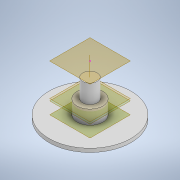
# Autodesk Inventor part: mold
Saved by Autodesk Inventor 2021 (Build 250183000, 183)
## iProperties
Created: 2020-07-07
Part Number: mold
Material: Generic
Document SubType Name: Modeling
Designer: adaml
Density: 1 g/cm^3
Appearance: Default
Author: adaml
Autodesk Inventor part; units mm, degrees
ref_plane "YZ Plane" through (0, 0, 0) normal (1, 0, 0) x (0, 1, 0)
ref_plane "XZ Plane" through (0, 0, 0) normal (0, 1, 0) x (-1, 0, 0)
ref_plane "XY Plane" through (0, 0, 0) normal (0, 0, 1) x (1, 0, 0)
ref_plane "Work Plane3" through (0, 0, 0) normal (0, -1, 0) x (1, 0, 0)
sketch "Sketch2" plane through (0, 0, 0) normal (0, -1, 0) x (1, 0, 0)
  circle A0 centre (0, 0) radius 22.352
  arc A1 (22.352, 0) -> (-22.352, 0) centre (0, 0) ccw projected
  line L0 (22.352, 0) -> (-22.352, 0)
  constraints: 2 end point, 1 centre point, 1 coincident, 1 horizontal
extrude "Extrusion2" add sketch "Sketch2" along normal blind 2
ref_plane "Work Plane5" through (0, 0, 0) normal (0, 1, 0) x (1, 0, 0)
sketch "Sketch3" plane through (0, 0, 0) normal (0, 1, 0) x (1, 0, 0)
  circle A0 centre (0, 0) radius 7
  line L0 (-20.955, 0) -> (20.955, 0) projected
  line L1 (-7, 0) -> (7, 0)
  dimension "d6" = 14
  constraints: 2 end point, 2 point on circle, 2 point on line, 1 centre point, 1 coincident
  measures "d6" diameter of A0
extrude "Extrusion3" add sketch "Sketch3" along normal blind 7.62
ref_plane "Work Plane4" through (0, -2, 0) normal (0, -1, 0) x (1, 0, 0)
sketch "Sketch4" plane through (0, -2, 0) normal (0, -1, 0) x (1, 0, 0)
  circle A0 centre (0, 0) radius 6
  dimension "d9" = 12
  constraints: 1 centre point, 1 coincident
  measures "d9" diameter of A0
extrude "Extrusion4" cut sketch "Sketch4" against normal blind 8.5725
ref_plane "Work Plane6" through (0, 7.62, 0) normal (0, 1, 0) x (1, 0, 0)
sketch "Sketch5" plane through (0, 7.62, 0) normal (0, 1, 0) x (1, 0, 0)
  circle A0 centre (0, 0) radius 4
  line L0 (7, 0) -> (-7, 0) projected
  line L1 (4, 0) -> (-4, 0)
  dimension "d12" = 8
  constraints: 2 end point, 2 point on circle, 2 point on line, 1 centre point, 1 coincident
  measures "d12" diameter of A0
extrude "Extrusion5" add sketch "Sketch5" along normal blind 10.16
ref_plane "Work Plane7" through (0, 6.5725, 0) normal (0, -1, 0) x (1, 0, 0)
sketch "Sketch6" plane through (0, 6.5725, 0) normal (0, -1, 0) x (1, 0, 0)
  circle A0 centre (0, 0) radius 3
  dimension "d15" = 6
  constraints: 1 centre point, 1 coincident
  measures "d15" diameter of A0
extrude "Extrusion6" cut sketch "Sketch6" against normal blind 10.16
ref_plane "Work Plane1" through (0, 25.4, 0) normal (0, 1, 0) x (1, 0, 0)
sketch "Sketch7" plane through (0, 25.4, 0) normal (0, 1, 0) x (1, 0, 0)
  point P0 (0, 0)
ref_plane "Work Plane2" through (0, 25.4, 0) normal (0, 1, 0) x (1, 0, 0)
sketch "Sketch12" plane through (0, 25.4, 0) normal (0, 1, 0) x (1, 0, 0)
  circle A0 centre (0, 0) radius 16.1182
  circle A1 centre (0, 0) radius 32.5204
  constraints: 2 centre point, 2 coincident
extrude "Extrusion10" cut sketch "Sketch12" against normal up to surface (25.4 mm away)
body "Solid1"
